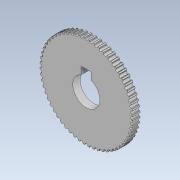
# Autodesk Inventor part: 2GT_60T
Saved by Autodesk Inventor 2022 (Build 260153000, 153)
## iProperties
Created: 2023-05-04
Part Number: 2GT_60T
Material: 一般
Document SubType Name: Modeling
Designer: Johnny Jou
Density: 1 g/cm^3
Appearance: 預設
Author: Johnny Jou
Autodesk Inventor part; units mm, degrees
ref_plane "YZ Plane" through (0, 0, 0) normal (1, 0, 0) x (0, 1, 0)
ref_plane "XZ Plane" through (0, 0, 0) normal (0, 1, 0) x (-1, 0, 0)
ref_plane "XY Plane" through (0, 0, 0) normal (0, 0, 1) x (1, 0, 0)
sketch "草圖1" plane through (0, 0, 0) normal (0, 0, 1) x (1, 0, 0)
  arc A0 (18.8049, -1.2283) -> (18.8303, -0.7441) centre (0, 0) ccw
  arc A1 (18.8303, -0.7441) -> (18.7019, -0.5897) centre (18.6804, -0.7382) ccw
  arc A2 (18.4068, -0.4989) -> (18.7019, -0.5897) centre (18.845, 0.4) ccw
  arc A3 (18.4068, 0.4989) -> (18.4068, -0.4989) centre (18.65, 0) ccw
  arc A4 (18.7019, 0.5897) -> (18.4068, 0.4989) centre (18.845, -0.4) ccw
  arc A5 (18.7019, 0.5897) -> (18.8303, 0.7441) centre (18.6804, 0.7382) ccw
  arc A6 (18.8303, 0.7441) -> (18.8049, 1.2283) centre (0, 0) ccw
  arc A7 (18.8049, 1.2283) -> (18.6611, 1.3684) centre (18.6552, 1.2185) ccw
  arc A8 (18.3581, 1.4279) -> (18.6611, 1.3684) centre (18.7, 2.3676) ccw
  arc A9 (18.2538, 2.4202) -> (18.3581, 1.4279) centre (18.5478, 1.9495) ccw
  arc A10 (18.5378, 2.5414) -> (18.2538, 2.4202) centre (18.7836, 1.572) ccw
  arc A11 (18.5378, 2.5414) -> (18.6494, 2.7083) centre (18.5009, 2.6868) ccw
  arc A12 (18.6494, 2.7083) -> (18.5735, 3.1872) centre (0, 0) ccw
  arc A13 (18.5735, 3.1872) -> (18.4158, 3.3115) centre (18.4257, 3.1618) ccw
  arc A14 (18.1083, 3.339) -> (18.4158, 3.3115) centre (18.35, 4.3094) ccw
  arc A15 (17.9008, 4.315) -> (18.1083, 3.339) centre (18.2425, 3.8776) ccw
  arc A16 (18.1706, 4.4652) -> (17.9008, 4.315) centre (18.5164, 3.5268) ccw
  arc A17 (18.1706, 4.4652) -> (18.2641, 4.6429) centre (18.1187, 4.6059) ccw
  arc A18 (18.2641, 4.6429) -> (18.1386, 5.1112) centre (0, 0) ccw
  arc A19 (18.1386, 5.1112) -> (17.9688, 5.2184) centre (17.9942, 5.0705) ccw
  arc A20 (17.6601, 5.2136) -> (17.9688, 5.2184) centre (17.7991, 6.2038) ccw
  arc A21 (17.3517, 6.1625) -> (17.6601, 5.2136) centre (17.7372, 5.7632) ccw
  arc A22 (17.6043, 6.34) -> (17.3517, 6.1625) centre (18.0463, 5.443) ccw
  arc A23 (17.6043, 6.34) -> (17.6787, 6.5266) centre (17.538, 6.4746) ccw
  arc A24 (17.6787, 6.5266) -> (17.505, 6.9792) centre (0, 0) ccw
  arc A25 (17.505, 6.9792) -> (17.3249, 7.068) centre (17.3657, 6.9237) ccw
  arc A26 (17.0184, 7.031) -> (17.3249, 7.068) centre (17.0531, 8.0304) ccw
  arc A27 (16.6125, 7.9425) -> (17.0184, 7.031) centre (17.0376, 7.5856) ccw
  arc A28 (16.8452, 8.1455) -> (16.6125, 7.9425) centre (17.3785, 7.2995) ccw
  arc A29 (16.8452, 8.1455) -> (16.8997, 8.3387) centre (16.7652, 8.2724) ccw
  arc A30 (16.8997, 8.3387) -> (16.6796, 8.7708) centre (0, 0) ccw
  arc A31 (16.6796, 8.7708) -> (16.4912, 8.8402) centre (16.5468, 8.7009) ccw
  arc A32 (16.1902, 8.7714) -> (16.4912, 8.8402) centre (16.1202, 9.7689) ccw
  arc A33 (15.6913, 9.6354) -> (16.1902, 8.7714) centre (16.1514, 9.325) ccw
  arc A34 (15.9015, 9.8616) -> (15.6913, 9.6354) centre (16.5202, 9.0761) ccw
  arc A35 (15.9015, 9.8616) -> (15.9355, 10.0595) centre (15.8086, 9.9795) ccw
  arc A36 (15.9355, 10.0595) -> (15.6714, 10.4662) centre (0, 0) ccw
  arc A37 (15.6714, 10.4662) -> (15.4768, 10.5156) centre (15.5467, 10.3829) ccw
  arc A38 (15.1846, 10.4156) -> (15.4768, 10.5156) centre (15.0108, 11.4004) ccw
  arc A39 (14.5982, 11.2228) -> (15.1846, 10.4156) centre (15.0882, 10.9622) ccw
  arc A40 (14.7835, 11.4698) -> (14.5982, 11.2228) centre (15.481, 10.7532) ccw
  arc A41 (14.7835, 11.4698) -> (14.7967, 11.6702) centre (14.6789, 11.5773) ccw
  arc A42 (14.7967, 11.6702) -> (14.4915, 12.047) centre (0, 0) ccw
  arc A43 (14.4915, 12.047) -> (14.2928, 12.0758) centre (14.3762, 11.9511) ccw
  arc A44 (14.0127, 11.9458) -> (14.2928, 12.0758) centre (13.7369, 12.907) ccw
  arc A45 (13.3451, 12.6873) -> (14.0127, 11.9458) centre (13.8597, 12.4793) ccw
  arc A46 (13.5036, 12.9522) -> (13.3451, 12.6873) centre (14.2722, 12.3125) ccw
  arc A47 (13.5036, 12.9522) -> (13.4958, 13.1529) centre (13.3883, 13.0482) ccw
  arc A48 (13.4958, 13.1529) -> (13.1529, 13.4958) centre (0, 0) ccw
  arc A49 (13.1529, 13.4958) -> (12.9522, 13.5036) centre (13.0482, 13.3883) ccw
  arc A50 (12.6873, 13.3451) -> (12.9522, 13.5036) centre (12.3125, 14.2722) ccw
  arc A51 (11.9458, 14.0127) -> (12.6873, 13.3451) centre (12.4793, 13.8597) ccw
  arc A52 (12.0758, 14.2928) -> (11.9458, 14.0127) centre (12.907, 13.7369) ccw
  arc A53 (12.0758, 14.2928) -> (12.047, 14.4915) centre (11.9511, 14.3762) ccw
  arc A54 (12.047, 14.4915) -> (11.6702, 14.7967) centre (0, 0) ccw
  arc A55 (11.6702, 14.7967) -> (11.4698, 14.7835) centre (11.5773, 14.6789) ccw
  arc A56 (11.2228, 14.5982) -> (11.4698, 14.7835) centre (10.7532, 15.481) ccw
  arc A57 (10.4156, 15.1846) -> (11.2228, 14.5982) centre (10.9622, 15.0882) ccw
  arc A58 (10.5156, 15.4768) -> (10.4156, 15.1846) centre (11.4004, 15.0108) ccw
  arc A59 (10.5156, 15.4768) -> (10.4662, 15.6714) centre (10.3829, 15.5467) ccw
  arc A60 (10.4662, 15.6714) -> (10.0595, 15.9355) centre (0, 0) ccw
  arc A61 (10.0595, 15.9355) -> (9.8616, 15.9015) centre (9.9795, 15.8086) ccw
  arc A62 (9.6354, 15.6913) -> (9.8616, 15.9015) centre (9.0761, 16.5202) ccw
  arc A63 (8.7714, 16.1902) -> (9.6354, 15.6913) centre (9.325, 16.1514) ccw
  arc A64 (8.8402, 16.4912) -> (8.7714, 16.1902) centre (9.7689, 16.1202) ccw
  arc A65 (8.8402, 16.4912) -> (8.7708, 16.6796) centre (8.7009, 16.5468) ccw
  arc A66 (8.7708, 16.6796) -> (8.3387, 16.8997) centre (0, 0) ccw
  arc A67 (8.3387, 16.8997) -> (8.1455, 16.8452) centre (8.2724, 16.7652) ccw
  arc A68 (7.9425, 16.6125) -> (8.1455, 16.8452) centre (7.2995, 17.3785) ccw
  arc A69 (7.031, 17.0184) -> (7.9425, 16.6125) centre (7.5856, 17.0376) ccw
  arc A70 (7.068, 17.3249) -> (7.031, 17.0184) centre (8.0304, 17.0531) ccw
  arc A71 (7.068, 17.3249) -> (6.9792, 17.505) centre (6.9237, 17.3657) ccw
  arc A72 (6.9792, 17.505) -> (6.5266, 17.6787) centre (0, 0) ccw
  arc A73 (6.5266, 17.6787) -> (6.34, 17.6043) centre (6.4746, 17.538) ccw
  arc A74 (6.1625, 17.3517) -> (6.34, 17.6043) centre (5.443, 18.0463) ccw
  arc A75 (5.2136, 17.6601) -> (6.1625, 17.3517) centre (5.7632, 17.7372) ccw
  arc A76 (5.2184, 17.9688) -> (5.2136, 17.6601) centre (6.2038, 17.7991) ccw
  arc A77 (5.2184, 17.9688) -> (5.1112, 18.1386) centre (5.0705, 17.9942) ccw
  arc A78 (5.1112, 18.1386) -> (4.6429, 18.2641) centre (0, 0) ccw
  arc A79 (4.6429, 18.2641) -> (4.4652, 18.1706) centre (4.6059, 18.1187) ccw
  arc A80 (4.315, 17.9008) -> (4.4652, 18.1706) centre (3.5268, 18.5164) ccw
  arc A81 (3.339, 18.1083) -> (4.315, 17.9008) centre (3.8776, 18.2425) ccw
  arc A82 (3.3115, 18.4158) -> (3.339, 18.1083) centre (4.3094, 18.35) ccw
  arc A83 (3.3115, 18.4158) -> (3.1872, 18.5735) centre (3.1618, 18.4257) ccw
  arc A84 (3.1872, 18.5735) -> (2.7083, 18.6494) centre (0, 0) ccw
  arc A85 (2.7083, 18.6494) -> (2.5414, 18.5378) centre (2.6868, 18.5009) ccw
  arc A86 (2.4202, 18.2538) -> (2.5414, 18.5378) centre (1.572, 18.7836) ccw
  arc A87 (1.4279, 18.3581) -> (2.4202, 18.2538) centre (1.9495, 18.5478) ccw
  arc A88 (1.3684, 18.6611) -> (1.4279, 18.3581) centre (2.3676, 18.7) ccw
  arc A89 (1.3684, 18.6611) -> (1.2283, 18.8049) centre (1.2185, 18.6552) ccw
  arc A90 (1.2283, 18.8049) -> (0.7441, 18.8303) centre (0, 0) ccw
  arc A91 (0.7441, 18.8303) -> (0.5897, 18.7019) centre (0.7382, 18.6804) ccw
  arc A92 (0.4989, 18.4068) -> (0.5897, 18.7019) centre (-0.4, 18.845) ccw
  arc A93 (-0.4989, 18.4068) -> (0.4989, 18.4068) centre (0, 18.65) ccw
  arc A94 (-0.5897, 18.7019) -> (-0.4989, 18.4068) centre (0.4, 18.845) ccw
  arc A95 (-0.5897, 18.7019) -> (-0.7441, 18.8303) centre (-0.7382, 18.6804) ccw
  arc A96 (-0.7441, 18.8303) -> (-1.2283, 18.8049) centre (0, 0) ccw
  arc A97 (-1.2283, 18.8049) -> (-1.3684, 18.6611) centre (-1.2185, 18.6552) ccw
  arc A98 (-1.4279, 18.3581) -> (-1.3684, 18.6611) centre (-2.3676, 18.7) ccw
  arc A99 (-2.4202, 18.2538) -> (-1.4279, 18.3581) centre (-1.9495, 18.5478) ccw
  arc A100 (-2.5414, 18.5378) -> (-2.4202, 18.2538) centre (-1.572, 18.7836) ccw
  arc A101 (-2.5414, 18.5378) -> (-2.7083, 18.6494) centre (-2.6868, 18.5009) ccw
  arc A102 (-2.7083, 18.6494) -> (-3.1872, 18.5735) centre (0, 0) ccw
  arc A103 (-3.1872, 18.5735) -> (-3.3115, 18.4158) centre (-3.1618, 18.4257) ccw
  arc A104 (-3.339, 18.1083) -> (-3.3115, 18.4158) centre (-4.3094, 18.35) ccw
  arc A105 (-4.315, 17.9008) -> (-3.339, 18.1083) centre (-3.8776, 18.2425) ccw
  arc A106 (-4.4652, 18.1706) -> (-4.315, 17.9008) centre (-3.5268, 18.5164) ccw
  arc A107 (-4.4652, 18.1706) -> (-4.6429, 18.2641) centre (-4.6059, 18.1187) ccw
  arc A108 (-4.6429, 18.2641) -> (-5.1112, 18.1386) centre (0, 0) ccw
  arc A109 (-5.1112, 18.1386) -> (-5.2184, 17.9688) centre (-5.0705, 17.9942) ccw
  arc A110 (-5.2136, 17.6601) -> (-5.2184, 17.9688) centre (-6.2038, 17.7991) ccw
  arc A111 (-6.1625, 17.3517) -> (-5.2136, 17.6601) centre (-5.7632, 17.7372) ccw
  arc A112 (-6.34, 17.6043) -> (-6.1625, 17.3517) centre (-5.443, 18.0463) ccw
  arc A113 (-6.34, 17.6043) -> (-6.5266, 17.6787) centre (-6.4746, 17.538) ccw
  arc A114 (-6.5266, 17.6787) -> (-6.9792, 17.505) centre (0, 0) ccw
  arc A115 (-6.9792, 17.505) -> (-7.068, 17.3249) centre (-6.9237, 17.3657) ccw
  arc A116 (-7.031, 17.0184) -> (-7.068, 17.3249) centre (-8.0304, 17.0531) ccw
  arc A117 (-7.9425, 16.6125) -> (-7.031, 17.0184) centre (-7.5856, 17.0376) ccw
  arc A118 (-8.1455, 16.8452) -> (-7.9425, 16.6125) centre (-7.2995, 17.3785) ccw
  arc A119 (-8.1455, 16.8452) -> (-8.3387, 16.8997) centre (-8.2724, 16.7652) ccw
  arc A120 (-8.3387, 16.8997) -> (-8.7708, 16.6796) centre (0, 0) ccw
  arc A121 (-8.7708, 16.6796) -> (-8.8402, 16.4912) centre (-8.7009, 16.5468) ccw
  arc A122 (-8.7714, 16.1902) -> (-8.8402, 16.4912) centre (-9.7689, 16.1202) ccw
  arc A123 (-9.6354, 15.6913) -> (-8.7714, 16.1902) centre (-9.325, 16.1514) ccw
  arc A124 (-9.8616, 15.9015) -> (-9.6354, 15.6913) centre (-9.0761, 16.5202) ccw
  arc A125 (-9.8616, 15.9015) -> (-10.0595, 15.9355) centre (-9.9795, 15.8086) ccw
  arc A126 (-10.0595, 15.9355) -> (-10.4662, 15.6714) centre (0, 0) ccw
  arc A127 (-10.4662, 15.6714) -> (-10.5156, 15.4768) centre (-10.3829, 15.5467) ccw
  arc A128 (-10.4156, 15.1846) -> (-10.5156, 15.4768) centre (-11.4004, 15.0108) ccw
  arc A129 (-11.2228, 14.5982) -> (-10.4156, 15.1846) centre (-10.9622, 15.0882) ccw
  arc A130 (-11.4698, 14.7835) -> (-11.2228, 14.5982) centre (-10.7532, 15.481) ccw
  arc A131 (-11.4698, 14.7835) -> (-11.6702, 14.7967) centre (-11.5773, 14.6789) ccw
  arc A132 (-11.6702, 14.7967) -> (-12.047, 14.4915) centre (0, 0) ccw
  arc A133 (-12.047, 14.4915) -> (-12.0758, 14.2928) centre (-11.9511, 14.3762) ccw
  arc A134 (-11.9458, 14.0127) -> (-12.0758, 14.2928) centre (-12.907, 13.7369) ccw
  arc A135 (-12.6873, 13.3451) -> (-11.9458, 14.0127) centre (-12.4793, 13.8597) ccw
  arc A136 (-12.9522, 13.5036) -> (-12.6873, 13.3451) centre (-12.3125, 14.2722) ccw
  arc A137 (-12.9522, 13.5036) -> (-13.1529, 13.4958) centre (-13.0482, 13.3883) ccw
  arc A138 (-13.1529, 13.4958) -> (-13.4958, 13.1529) centre (0, 0) ccw
  arc A139 (-13.4958, 13.1529) -> (-13.5036, 12.9522) centre (-13.3883, 13.0482) ccw
  arc A140 (-13.3451, 12.6873) -> (-13.5036, 12.9522) centre (-14.2722, 12.3125) ccw
  arc A141 (-14.0127, 11.9458) -> (-13.3451, 12.6873) centre (-13.8597, 12.4793) ccw
  arc A142 (-14.2928, 12.0758) -> (-14.0127, 11.9458) centre (-13.7369, 12.907) ccw
  arc A143 (-14.2928, 12.0758) -> (-14.4915, 12.047) centre (-14.3762, 11.9511) ccw
  arc A144 (-14.4915, 12.047) -> (-14.7967, 11.6702) centre (0, 0) ccw
  arc A145 (-14.7967, 11.6702) -> (-14.7835, 11.4698) centre (-14.6789, 11.5773) ccw
  arc A146 (-14.5982, 11.2228) -> (-14.7835, 11.4698) centre (-15.481, 10.7532) ccw
  arc A147 (-15.1846, 10.4156) -> (-14.5982, 11.2228) centre (-15.0882, 10.9622) ccw
  arc A148 (-15.4768, 10.5156) -> (-15.1846, 10.4156) centre (-15.0108, 11.4004) ccw
  arc A149 (-15.4768, 10.5156) -> (-15.6714, 10.4662) centre (-15.5467, 10.3829) ccw
  arc A150 (-15.6714, 10.4662) -> (-15.9355, 10.0595) centre (0, 0) ccw
  arc A151 (-15.9355, 10.0595) -> (-15.9015, 9.8616) centre (-15.8086, 9.9795) ccw
  arc A152 (-15.6913, 9.6354) -> (-15.9015, 9.8616) centre (-16.5202, 9.0761) ccw
  arc A153 (-16.1902, 8.7714) -> (-15.6913, 9.6354) centre (-16.1514, 9.325) ccw
  arc A154 (-16.4912, 8.8402) -> (-16.1902, 8.7714) centre (-16.1202, 9.7689) ccw
  arc A155 (-16.4912, 8.8402) -> (-16.6796, 8.7708) centre (-16.5468, 8.7009) ccw
  arc A156 (-16.6796, 8.7708) -> (-16.8997, 8.3387) centre (0, 0) ccw
  arc A157 (-16.8997, 8.3387) -> (-16.8452, 8.1455) centre (-16.7652, 8.2724) ccw
  arc A158 (-16.6125, 7.9425) -> (-16.8452, 8.1455) centre (-17.3785, 7.2995) ccw
  arc A159 (-17.0184, 7.031) -> (-16.6125, 7.9425) centre (-17.0376, 7.5856) ccw
  arc A160 (-17.3249, 7.068) -> (-17.0184, 7.031) centre (-17.0531, 8.0304) ccw
  arc A161 (-17.3249, 7.068) -> (-17.505, 6.9792) centre (-17.3657, 6.9237) ccw
  arc A162 (-17.505, 6.9792) -> (-17.6787, 6.5266) centre (0, 0) ccw
  arc A163 (-17.6787, 6.5266) -> (-17.6043, 6.34) centre (-17.538, 6.4746) ccw
  arc A164 (-17.3517, 6.1625) -> (-17.6043, 6.34) centre (-18.0463, 5.443) ccw
  arc A165 (-17.6601, 5.2136) -> (-17.3517, 6.1625) centre (-17.7372, 5.7632) ccw
  arc A166 (-17.9688, 5.2184) -> (-17.6601, 5.2136) centre (-17.7991, 6.2038) ccw
  arc A167 (-17.9688, 5.2184) -> (-18.1386, 5.1112) centre (-17.9942, 5.0705) ccw
  arc A168 (-18.1386, 5.1112) -> (-18.2641, 4.6429) centre (0, 0) ccw
  arc A169 (-18.2641, 4.6429) -> (-18.1706, 4.4652) centre (-18.1187, 4.6059) ccw
  arc A170 (-17.9008, 4.315) -> (-18.1706, 4.4652) centre (-18.5164, 3.5268) ccw
  arc A171 (-18.1083, 3.339) -> (-17.9008, 4.315) centre (-18.2425, 3.8776) ccw
  arc A172 (-18.4158, 3.3115) -> (-18.1083, 3.339) centre (-18.35, 4.3094) ccw
  arc A173 (-18.4158, 3.3115) -> (-18.5735, 3.1872) centre (-18.4257, 3.1618) ccw
  arc A174 (-18.5735, 3.1872) -> (-18.6494, 2.7083) centre (0, 0) ccw
  arc A175 (-18.6494, 2.7083) -> (-18.5378, 2.5414) centre (-18.5009, 2.6868) ccw
  arc A176 (-18.2538, 2.4202) -> (-18.5378, 2.5414) centre (-18.7836, 1.572) ccw
  arc A177 (-18.3581, 1.4279) -> (-18.2538, 2.4202) centre (-18.5478, 1.9495) ccw
  arc A178 (-18.6611, 1.3684) -> (-18.3581, 1.4279) centre (-18.7, 2.3676) ccw
  arc A179 (-18.6611, 1.3684) -> (-18.8049, 1.2283) centre (-18.6552, 1.2185) ccw
  arc A180 (-18.8049, 1.2283) -> (-18.8303, 0.7441) centre (0, 0) ccw
  arc A181 (-18.8303, 0.7441) -> (-18.7019, 0.5897) centre (-18.6804, 0.7382) ccw
  arc A182 (-18.4068, 0.4989) -> (-18.7019, 0.5897) centre (-18.845, -0.4) ccw
  arc A183 (-18.4068, -0.4989) -> (-18.4068, 0.4989) centre (-18.65, 0) ccw
  arc A184 (-18.7019, -0.5897) -> (-18.4068, -0.4989) centre (-18.845, 0.4) ccw
  arc A185 (-18.7019, -0.5897) -> (-18.8303, -0.7441) centre (-18.6804, -0.7382) ccw
  arc A186 (-18.8303, -0.7441) -> (-18.8049, -1.2283) centre (0, 0) ccw
  arc A187 (-18.8049, -1.2283) -> (-18.6611, -1.3684) centre (-18.6552, -1.2185) ccw
  arc A188 (-18.3581, -1.4279) -> (-18.6611, -1.3684) centre (-18.7, -2.3676) ccw
  arc A189 (-18.2538, -2.4202) -> (-18.3581, -1.4279) centre (-18.5478, -1.9495) ccw
  arc A190 (-18.5378, -2.5414) -> (-18.2538, -2.4202) centre (-18.7836, -1.572) ccw
  arc A191 (-18.5378, -2.5414) -> (-18.6494, -2.7083) centre (-18.5009, -2.6868) ccw
  arc A192 (-18.6494, -2.7083) -> (-18.5735, -3.1872) centre (0, 0) ccw
  arc A193 (-18.5735, -3.1872) -> (-18.4158, -3.3115) centre (-18.4257, -3.1618) ccw
  arc A194 (-18.1083, -3.339) -> (-18.4158, -3.3115) centre (-18.35, -4.3094) ccw
  arc A195 (-17.9008, -4.315) -> (-18.1083, -3.339) centre (-18.2425, -3.8776) ccw
  arc A196 (-18.1706, -4.4652) -> (-17.9008, -4.315) centre (-18.5164, -3.5268) ccw
  arc A197 (-18.1706, -4.4652) -> (-18.2641, -4.6429) centre (-18.1187, -4.6059) ccw
  arc A198 (-18.2641, -4.6429) -> (-18.1386, -5.1112) centre (0, 0) ccw
  arc A199 (-18.1386, -5.1112) -> (-17.9688, -5.2184) centre (-17.9942, -5.0705) ccw
  arc A200 (-17.6601, -5.2136) -> (-17.9688, -5.2184) centre (-17.7991, -6.2038) ccw
  arc A201 (-17.3517, -6.1625) -> (-17.6601, -5.2136) centre (-17.7372, -5.7632) ccw
  arc A202 (-17.6043, -6.34) -> (-17.3517, -6.1625) centre (-18.0463, -5.443) ccw
  arc A203 (-17.6043, -6.34) -> (-17.6787, -6.5266) centre (-17.538, -6.4746) ccw
  arc A204 (-17.6787, -6.5266) -> (-17.505, -6.9792) centre (0, 0) ccw
  arc A205 (-17.505, -6.9792) -> (-17.3249, -7.068) centre (-17.3657, -6.9237) ccw
  arc A206 (-17.0184, -7.031) -> (-17.3249, -7.068) centre (-17.0531, -8.0304) ccw
  arc A207 (-16.6125, -7.9425) -> (-17.0184, -7.031) centre (-17.0376, -7.5856) ccw
  arc A208 (-16.8452, -8.1455) -> (-16.6125, -7.9425) centre (-17.3785, -7.2995) ccw
  arc A209 (-16.8452, -8.1455) -> (-16.8997, -8.3387) centre (-16.7652, -8.2724) ccw
  arc A210 (-16.8997, -8.3387) -> (-16.6796, -8.7708) centre (0, 0) ccw
  arc A211 (-16.6796, -8.7708) -> (-16.4912, -8.8402) centre (-16.5468, -8.7009) ccw
  arc A212 (-16.1902, -8.7714) -> (-16.4912, -8.8402) centre (-16.1202, -9.7689) ccw
  arc A213 (-15.6913, -9.6354) -> (-16.1902, -8.7714) centre (-16.1514, -9.325) ccw
  arc A214 (-15.9015, -9.8616) -> (-15.6913, -9.6354) centre (-16.5202, -9.0761) ccw
  arc A215 (-15.9015, -9.8616) -> (-15.9355, -10.0595) centre (-15.8086, -9.9795) ccw
  arc A216 (-15.9355, -10.0595) -> (-15.6714, -10.4662) centre (0, 0) ccw
  arc A217 (-15.6714, -10.4662) -> (-15.4768, -10.5156) centre (-15.5467, -10.3829) ccw
  arc A218 (-15.1846, -10.4156) -> (-15.4768, -10.5156) centre (-15.0108, -11.4004) ccw
  arc A219 (-14.5982, -11.2228) -> (-15.1846, -10.4156) centre (-15.0882, -10.9622) ccw
  arc A220 (-14.7835, -11.4698) -> (-14.5982, -11.2228) centre (-15.481, -10.7532) ccw
  arc A221 (-14.7835, -11.4698) -> (-14.7967, -11.6702) centre (-14.6789, -11.5773) ccw
  arc A222 (-14.7967, -11.6702) -> (-14.4915, -12.047) centre (0, 0) ccw
  arc A223 (-14.4915, -12.047) -> (-14.2928, -12.0758) centre (-14.3762, -11.9511) ccw
  arc A224 (-14.0127, -11.9458) -> (-14.2928, -12.0758) centre (-13.7369, -12.907) ccw
  arc A225 (-13.3451, -12.6873) -> (-14.0127, -11.9458) centre (-13.8597, -12.4793) ccw
  arc A226 (-13.5036, -12.9522) -> (-13.3451, -12.6873) centre (-14.2722, -12.3125) ccw
  arc A227 (-13.5036, -12.9522) -> (-13.4958, -13.1529) centre (-13.3883, -13.0482) ccw
  arc A228 (-13.4958, -13.1529) -> (-13.1529, -13.4958) centre (0, 0) ccw
  arc A229 (-13.1529, -13.4958) -> (-12.9522, -13.5036) centre (-13.0482, -13.3883) ccw
  arc A230 (-12.6873, -13.3451) -> (-12.9522, -13.5036) centre (-12.3125, -14.2722) ccw
  arc A231 (-11.9458, -14.0127) -> (-12.6873, -13.3451) centre (-12.4793, -13.8597) ccw
  arc A232 (-12.0758, -14.2928) -> (-11.9458, -14.0127) centre (-12.907, -13.7369) ccw
  arc A233 (-12.0758, -14.2928) -> (-12.047, -14.4915) centre (-11.9511, -14.3762) ccw
  arc A234 (-12.047, -14.4915) -> (-11.6702, -14.7967) centre (0, 0) ccw
  arc A235 (-11.6702, -14.7967) -> (-11.4698, -14.7835) centre (-11.5773, -14.6789) ccw
  arc A236 (-11.2228, -14.5982) -> (-11.4698, -14.7835) centre (-10.7532, -15.481) ccw
  arc A237 (-10.4156, -15.1846) -> (-11.2228, -14.5982) centre (-10.9622, -15.0882) ccw
  arc A238 (-10.5156, -15.4768) -> (-10.4156, -15.1846) centre (-11.4004, -15.0108) ccw
  arc A239 (-10.5156, -15.4768) -> (-10.4662, -15.6714) centre (-10.3829, -15.5467) ccw
  arc A240 (-10.4662, -15.6714) -> (-10.0595, -15.9355) centre (0, 0) ccw
  arc A241 (-10.0595, -15.9355) -> (-9.8616, -15.9015) centre (-9.9795, -15.8086) ccw
  arc A242 (-9.6354, -15.6913) -> (-9.8616, -15.9015) centre (-9.0761, -16.5202) ccw
  arc A243 (-8.7714, -16.1902) -> (-9.6354, -15.6913) centre (-9.325, -16.1514) ccw
  arc A244 (-8.8402, -16.4912) -> (-8.7714, -16.1902) centre (-9.7689, -16.1202) ccw
  arc A245 (-8.8402, -16.4912) -> (-8.7708, -16.6796) centre (-8.7009, -16.5468) ccw
  arc A246 (-8.7708, -16.6796) -> (-8.3387, -16.8997) centre (0, 0) ccw
  arc A247 (-8.3387, -16.8997) -> (-8.1455, -16.8452) centre (-8.2724, -16.7652) ccw
  arc A248 (-7.9425, -16.6125) -> (-8.1455, -16.8452) centre (-7.2995, -17.3785) ccw
  arc A249 (-7.031, -17.0184) -> (-7.9425, -16.6125) centre (-7.5856, -17.0376) ccw
  arc A250 (-7.068, -17.3249) -> (-7.031, -17.0184) centre (-8.0304, -17.0531) ccw
  arc A251 (-7.068, -17.3249) -> (-6.9792, -17.505) centre (-6.9237, -17.3657) ccw
  arc A252 (-6.9792, -17.505) -> (-6.5266, -17.6787) centre (0, 0) ccw
  arc A253 (-6.5266, -17.6787) -> (-6.34, -17.6043) centre (-6.4746, -17.538) ccw
  arc A254 (-6.1625, -17.3517) -> (-6.34, -17.6043) centre (-5.443, -18.0463) ccw
  arc A255 (-5.2136, -17.6601) -> (-6.1625, -17.3517) centre (-5.7632, -17.7372) ccw
  arc A256 (-5.2184, -17.9688) -> (-5.2136, -17.6601) centre (-6.2038, -17.7991) ccw
  arc A257 (-5.2184, -17.9688) -> (-5.1112, -18.1386) centre (-5.0705, -17.9942) ccw
  arc A258 (-5.1112, -18.1386) -> (-4.6429, -18.2641) centre (0, 0) ccw
  arc A259 (-4.6429, -18.2641) -> (-4.4652, -18.1706) centre (-4.6059, -18.1187) ccw
  arc A260 (-4.315, -17.9008) -> (-4.4652, -18.1706) centre (-3.5268, -18.5164) ccw
  arc A261 (-3.339, -18.1083) -> (-4.315, -17.9008) centre (-3.8776, -18.2425) ccw
  arc A262 (-3.3115, -18.4158) -> (-3.339, -18.1083) centre (-4.3094, -18.35) ccw
  arc A263 (-3.3115, -18.4158) -> (-3.1872, -18.5735) centre (-3.1618, -18.4257) ccw
  arc A264 (-3.1872, -18.5735) -> (-2.7083, -18.6494) centre (0, 0) ccw
  arc A265 (-2.7083, -18.6494) -> (-2.5414, -18.5378) centre (-2.6868, -18.5009) ccw
  arc A266 (-2.4202, -18.2538) -> (-2.5414, -18.5378) centre (-1.572, -18.7836) ccw
  arc A267 (-1.4279, -18.3581) -> (-2.4202, -18.2538) centre (-1.9495, -18.5478) ccw
  arc A268 (-1.3684, -18.6611) -> (-1.4279, -18.3581) centre (-2.3676, -18.7) ccw
  arc A269 (-1.3684, -18.6611) -> (-1.2283, -18.8049) centre (-1.2185, -18.6552) ccw
  arc A270 (-1.2283, -18.8049) -> (-0.7441, -18.8303) centre (0, 0) ccw
  arc A271 (-0.7441, -18.8303) -> (-0.5897, -18.7019) centre (-0.7382, -18.6804) ccw
  arc A272 (-0.4989, -18.4068) -> (-0.5897, -18.7019) centre (0.4, -18.845) ccw
  arc A273 (0.4989, -18.4068) -> (-0.4989, -18.4068) centre (0, -18.65) ccw
  arc A274 (0.5897, -18.7019) -> (0.4989, -18.4068) centre (-0.4, -18.845) ccw
  arc A275 (0.5897, -18.7019) -> (0.7441, -18.8303) centre (0.7382, -18.6804) ccw
  arc A276 (0.7441, -18.8303) -> (1.2283, -18.8049) centre (0, 0) ccw
  arc A277 (1.2283, -18.8049) -> (1.3684, -18.6611) centre (1.2185, -18.6552) ccw
  arc A278 (1.4279, -18.3581) -> (1.3684, -18.6611) centre (2.3676, -18.7) ccw
  arc A279 (2.4202, -18.2538) -> (1.4279, -18.3581) centre (1.9495, -18.5478) ccw
  arc A280 (2.5414, -18.5378) -> (2.4202, -18.2538) centre (1.572, -18.7836) ccw
  arc A281 (2.5414, -18.5378) -> (2.7083, -18.6494) centre (2.6868, -18.5009) ccw
  arc A282 (2.7083, -18.6494) -> (3.1872, -18.5735) centre (0, 0) ccw
  arc A283 (3.1872, -18.5735) -> (3.3115, -18.4158) centre (3.1618, -18.4257) ccw
  arc A284 (3.339, -18.1083) -> (3.3115, -18.4158) centre (4.3094, -18.35) ccw
  arc A285 (4.315, -17.9008) -> (3.339, -18.1083) centre (3.8776, -18.2425) ccw
  arc A286 (4.4652, -18.1706) -> (4.315, -17.9008) centre (3.5268, -18.5164) ccw
  arc A287 (4.4652, -18.1706) -> (4.6429, -18.2641) centre (4.6059, -18.1187) ccw
  arc A288 (4.6429, -18.2641) -> (5.1112, -18.1386) centre (0, 0) ccw
  arc A289 (5.1112, -18.1386) -> (5.2184, -17.9688) centre (5.0705, -17.9942) ccw
  arc A290 (5.2136, -17.6601) -> (5.2184, -17.9688) centre (6.2038, -17.7991) ccw
  arc A291 (6.1625, -17.3517) -> (5.2136, -17.6601) centre (5.7632, -17.7372) ccw
  arc A292 (6.34, -17.6043) -> (6.1625, -17.3517) centre (5.443, -18.0463) ccw
  arc A293 (6.34, -17.6043) -> (6.5266, -17.6787) centre (6.4746, -17.538) ccw
  arc A294 (6.5266, -17.6787) -> (6.9792, -17.505) centre (0, 0) ccw
  arc A295 (6.9792, -17.505) -> (7.068, -17.3249) centre (6.9237, -17.3657) ccw
  arc A296 (7.031, -17.0184) -> (7.068, -17.3249) centre (8.0304, -17.0531) ccw
  arc A297 (7.9425, -16.6125) -> (7.031, -17.0184) centre (7.5856, -17.0376) ccw
  arc A298 (8.1455, -16.8452) -> (7.9425, -16.6125) centre (7.2995, -17.3785) ccw
  arc A299 (8.1455, -16.8452) -> (8.3387, -16.8997) centre (8.2724, -16.7652) ccw
  arc A300 (8.3387, -16.8997) -> (8.7708, -16.6796) centre (0, 0) ccw
  arc A301 (8.7708, -16.6796) -> (8.8402, -16.4912) centre (8.7009, -16.5468) ccw
  arc A302 (8.7714, -16.1902) -> (8.8402, -16.4912) centre (9.7689, -16.1202) ccw
  arc A303 (9.6354, -15.6913) -> (8.7714, -16.1902) centre (9.325, -16.1514) ccw
  arc A304 (9.8616, -15.9015) -> (9.6354, -15.6913) centre (9.0761, -16.5202) ccw
  arc A305 (9.8616, -15.9015) -> (10.0595, -15.9355) centre (9.9795, -15.8086) ccw
  arc A306 (10.0595, -15.9355) -> (10.4662, -15.6714) centre (0, 0) ccw
  arc A307 (10.4662, -15.6714) -> (10.5156, -15.4768) centre (10.3829, -15.5467) ccw
  arc A308 (10.4156, -15.1846) -> (10.5156, -15.4768) centre (11.4004, -15.0108) ccw
  arc A309 (11.2228, -14.5982) -> (10.4156, -15.1846) centre (10.9622, -15.0882) ccw
  arc A310 (11.4698, -14.7835) -> (11.2228, -14.5982) centre (10.7532, -15.481) ccw
  arc A311 (11.4698, -14.7835) -> (11.6702, -14.7967) centre (11.5773, -14.6789) ccw
  arc A312 (11.6702, -14.7967) -> (12.047, -14.4915) centre (0, 0) ccw
  arc A313 (12.047, -14.4915) -> (12.0758, -14.2928) centre (11.9511, -14.3762) ccw
  arc A314 (11.9458, -14.0127) -> (12.0758, -14.2928) centre (12.907, -13.7369) ccw
  arc A315 (12.6873, -13.3451) -> (11.9458, -14.0127) centre (12.4793, -13.8597) ccw
  arc A316 (12.9522, -13.5036) -> (12.6873, -13.3451) centre (12.3125, -14.2722) ccw
  arc A317 (12.9522, -13.5036) -> (13.1529, -13.4958) centre (13.0482, -13.3883) ccw
  arc A318 (13.1529, -13.4958) -> (13.4958, -13.1529) centre (0, 0) ccw
  arc A319 (13.4958, -13.1529) -> (13.5036, -12.9522) centre (13.3883, -13.0482) ccw
  arc A320 (13.3451, -12.6873) -> (13.5036, -12.9522) centre (14.2722, -12.3125) ccw
  arc A321 (14.0127, -11.9458) -> (13.3451, -12.6873) centre (13.8597, -12.4793) ccw
  arc A322 (14.2928, -12.0758) -> (14.0127, -11.9458) centre (13.7369, -12.907) ccw
  arc A323 (14.2928, -12.0758) -> (14.4915, -12.047) centre (14.3762, -11.9511) ccw
  arc A324 (14.4915, -12.047) -> (14.7967, -11.6702) centre (0, 0) ccw
  arc A325 (14.7967, -11.6702) -> (14.7835, -11.4698) centre (14.6789, -11.5773) ccw
  arc A326 (14.5982, -11.2228) -> (14.7835, -11.4698) centre (15.481, -10.7532) ccw
  arc A327 (15.1846, -10.4156) -> (14.5982, -11.2228) centre (15.0882, -10.9622) ccw
  arc A328 (15.4768, -10.5156) -> (15.1846, -10.4156) centre (15.0108, -11.4004) ccw
  arc A329 (15.4768, -10.5156) -> (15.6714, -10.4662) centre (15.5467, -10.3829) ccw
  arc A330 (15.6714, -10.4662) -> (15.9355, -10.0595) centre (0, 0) ccw
  arc A331 (15.9355, -10.0595) -> (15.9015, -9.8616) centre (15.8086, -9.9795) ccw
  arc A332 (15.6913, -9.6354) -> (15.9015, -9.8616) centre (16.5202, -9.0761) ccw
  arc A333 (16.1902, -8.7714) -> (15.6913, -9.6354) centre (16.1514, -9.325) ccw
  arc A334 (16.4912, -8.8402) -> (16.1902, -8.7714) centre (16.1202, -9.7689) ccw
  arc A335 (16.4912, -8.8402) -> (16.6796, -8.7708) centre (16.5468, -8.7009) ccw
  arc A336 (16.6796, -8.7708) -> (16.8997, -8.3387) centre (0, 0) ccw
  arc A337 (16.8997, -8.3387) -> (16.8452, -8.1455) centre (16.7652, -8.2724) ccw
  arc A338 (16.6125, -7.9425) -> (16.8452, -8.1455) centre (17.3785, -7.2995) ccw
  arc A339 (17.0184, -7.031) -> (16.6125, -7.9425) centre (17.0376, -7.5856) ccw
  arc A340 (17.3249, -7.068) -> (17.0184, -7.031) centre (17.0531, -8.0304) ccw
  arc A341 (17.3249, -7.068) -> (17.505, -6.9792) centre (17.3657, -6.9237) ccw
  arc A342 (17.505, -6.9792) -> (17.6787, -6.5266) centre (0, 0) ccw
  arc A343 (17.6787, -6.5266) -> (17.6043, -6.34) centre (17.538, -6.4746) ccw
  arc A344 (17.3517, -6.1625) -> (17.6043, -6.34) centre (18.0463, -5.443) ccw
  arc A345 (17.6601, -5.2136) -> (17.3517, -6.1625) centre (17.7372, -5.7632) ccw
  arc A346 (17.9688, -5.2184) -> (17.6601, -5.2136) centre (17.7991, -6.2038) ccw
  arc A347 (17.9688, -5.2184) -> (18.1386, -5.1112) centre (17.9942, -5.0705) ccw
  arc A348 (18.1386, -5.1112) -> (18.2641, -4.6429) centre (0, 0) ccw
  arc A349 (18.2641, -4.6429) -> (18.1706, -4.4652) centre (18.1187, -4.6059) ccw
  arc A350 (17.9008, -4.315) -> (18.1706, -4.4652) centre (18.5164, -3.5268) ccw
  arc A351 (18.1083, -3.339) -> (17.9008, -4.315) centre (18.2425, -3.8776) ccw
  arc A352 (18.4158, -3.3115) -> (18.1083, -3.339) centre (18.35, -4.3094) ccw
  arc A353 (18.4158, -3.3115) -> (18.5735, -3.1872) centre (18.4257, -3.1618) ccw
  arc A354 (18.5735, -3.1872) -> (18.6494, -2.7083) centre (0, 0) ccw
  arc A355 (18.6494, -2.7083) -> (18.5378, -2.5414) centre (18.5009, -2.6868) ccw
  arc A356 (18.2538, -2.4202) -> (18.5378, -2.5414) centre (18.7836, -1.572) ccw
  arc A357 (18.3581, -1.4279) -> (18.2538, -2.4202) centre (18.5478, -1.9495) ccw
  arc A358 (18.6611, -1.3684) -> (18.3581, -1.4279) centre (18.7, -2.3676) ccw
  arc A359 (18.6611, -1.3684) -> (18.8049, -1.2283) centre (18.6552, -1.2185) ccw
  circle A360 centre (0, 0) radius 5.5
  line L0 (-2, 8.1235) -> (2, 8.1235)
  line L1 (2, 8.1235) -> (2, 5.1235)
  line L2 (2, 5.1235) -> (-2, 5.1235)
  line L3 (-2, 5.1235) -> (-2, 8.1235)
  dimension "d0" = 11
  dimension "d1" = 3
  dimension "d2" = 4
  constraints: 722 point on circle, 361 centre point, 8 end point, 2 parallel, 1 coincident, 1 horizontal, 1 perpendicular, 1020 other
  measures "d0" diameter of A360
  measures "d1" distance of L0.end L1.end
  measures "d2" distance of L0.start L0.end
extrude "擠出1" add sketch "草圖1" along normal blind 3
